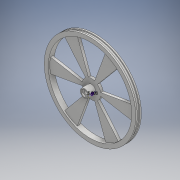
# Autodesk Inventor part: smallWheel
Saved by Autodesk Inventor 2018 (Build 220112000, 112)
## iProperties
Created: 2017-10-25
Part Number: smallWheel
Material: Generic
Document SubType Name: Modeling
Designer: Payal Jindal
Density: 1 g/cm^3
Appearance: Default
Author: Payal Jindal
Autodesk Inventor part; units mm, degrees
ref_plane "XZ Plane" through (0, 0, 0) normal (0, 1, 0) x (-1, 0, 0)
ref_plane "XY Plane" through (0, 0, 0) normal (0, 0, 1) x (1, 0, 0)
sketch "Sketch1" plane through (0, 0, 0) normal (0, 1, 0) x (-1, 0, 0)
  circle A0 centre (0, 0) radius 90
  circle A1 centre (0, 0) radius 88
  circle A2 centre (0, 0) radius 82
  circle A3 centre (0, 0) radius 3.175
  circle A4 centre (0, 0) radius 8.175
  circle A5 centre (0, 0) radius 18.175
  line L0 (0, 0) -> (28.0457, 77.0548)
  line L1 (0, 0) -> (-28.0457, 77.0548)
  line L2 (0, 0) -> (0, 82)
  arc A6 (6.2162, 17.0789) -> (-6.2162, 17.0789) centre (0, 0) ccw
  dimension "d0" = 180
  dimension "d3" = 2
  dimension "d6" = 8
  dimension "d11" = 6.35
  dimension "d14" = 5
  dimension "d35" = 10
  dimension "d60" = 20
  dimension "d61" = 20
  constraints: 7 centre point, 7 coincident, 7 point on circle, 6 end point, 2 point on line, 1 vertical
  measures "d0" diameter of A0
  measures "d3" radial gap between concentric circles of A0 A1
  measures "d6" radial gap between concentric circles of A2 A0
  measures "d11" diameter of A3
  measures "d14" radial gap between concentric circles of A4 A3
  measures "d35" radial gap between concentric circles of A4 A5
  measures "d60" angle of L1 L2
  measures "d61" angle of L2 L0
extrude "Extrusion2" add sketch "Sketch1" along normal blind 5 contours A1 | A2 L1 A5 L0 | L0 A5 L2 A2 | A2 L2 A5 L1 | L0 A4 L2 A5 | A5 L1 A4 L0 | A5 L2 A4 L1 | L0 A3 L2 A4 | A4 L1 A3 L0 | A4 L2 A3 L1 | L0 L2 A3 | A3 L1 L0 | A3 L2 L1
extrude "Extrusion3" add sketch "Sketch1" against normal blind 3 contours A0 | A1
sketch "Sketch3" plane through (0, 5, 0) normal (0, 1, 0) x (1, 0, 0)
  circle A0 centre (0, 0) radius 82 projected
  circle A1 centre (0, 0) radius 90 projected
extrude "Extrusion4" add sketch "Sketch3" along normal blind 3
extrude "Extrusion5" cut sketch "Sketch1" along normal blind 35.75 contours L0 L2 A3 | A3 L1 L0 | A3 L2 L1
extrude "Extrusion6" add sketch "Sketch1" against normal blind 14 contours L0 A3 L2 A4 | A4 L1 A3 L0 | A4 L2 A3 L1
ref_plane "Work Plane1" through (8.175, 0, 0) normal (1, 0, 0) x (0, 1, 0)
sketch "Sketch5" plane through (8.175, 0, 0) normal (1, 0, 0) x (0, 1, 0)
  line L0 (-14, -3.175) -> (-14, 3.175) construction
  line L1 (-14, 0) -> (0, 0) construction
  circle A0 centre (-7, 0) radius 2.6543
  circle A1 centre (-7, 0) radius 2.5273
  dimension "d49" = 5.3086
  dimension "d50" = 5.0546
  constraints: 2 centre point, 2 end point, 2 midpoint, 1 coincident, 1 horizontal
  measures "d49" diameter of A0
  measures "d50" diameter of A1
extrude "Extrusion9" cut sketch "Sketch5" against normal blind 3.81 contours A1
loft "Loft1" cut profiles "Sketch5" section 2 edges at (4.365, -9.5273, 0) contours A0 | A1
sketch "Sketch6" plane through (0, -14, 0) normal (0, -1, 0) x (1, 0, 0)
  line L0 (-6.0562, 3.4966) -> (0, 6.9932)
  line L1 (0, 6.9932) -> (6.0562, 3.4966)
  line L2 (6.0562, 3.4966) -> (6.0562, -3.4966)
  line L3 (6.0562, -3.4966) -> (0, -6.9932)
  line L4 (0, -6.9932) -> (-6.0562, -3.4966)
  line L5 (-6.0562, -3.4966) -> (-6.0562, 3.4966)
  point P0 (0, 0)
  point P1 (0, 0)
  dimension "d57" = 12.1125
  constraints: 12 end point, 1 coincident, 1 vertical, 13 other
  measures "d57" distance between parallel lines of L5 L2
extrude "Extrusion10" cut sketch "Sketch6" against normal blind 3
extrude "Extrusion11" cut sketch "Sketch1" along normal up to surface (5 mm away) contours L0 A5 L2 A2 | A2 L2 A5 L1
pattern_circular "Circular Pattern1" count 6 over 360 about axis through (0, 0, 0) along (0, -1, 0) of "Extrusion11"
sketch "Sketch7" plane through (0, 5, 0) normal (0, 1, 0) x (1, 0, 0)
  circle A0 centre (0, 0) radius 13
  dimension "d67" = 26
  constraints: 1 centre point, 1 coincident
  measures "d67" diameter of A0
extrude "Extrusion12" cut sketch "Sketch7" against normal blind 2
equation "\"d61\" = d60"
body "Solid2"
